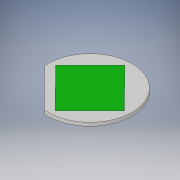
# Autodesk Inventor part: RockSat Plate
Saved by Autodesk Inventor 2017 (Build 210142000, 142)
## iProperties
Created: 2016-12-06
Part Number: RockSat Plate
Material: Generic
Document SubType Name: Modeling
Designer: qupec
Density: 1 g/cm^3
Appearance: Default
Author: qupec
Autodesk Inventor part; units mm, degrees
ref_plane "YZ Plane" through (0, 0, 0) normal (1, 0, 0) x (0, 1, 0)
ref_plane "XZ Plane" through (0, 0, 0) normal (0, 1, 0) x (-1, 0, 0)
ref_plane "XY Plane" through (0, 0, 0) normal (0, 0, 1) x (1, 0, 0)
sketch "Sketch1" plane through (0, 0, 0) normal (0, 1, 0) x (-1, 0, 0)
  arc A0 (13.4296, 151.8071) -> (151.8071, 13.4296) centre (0, 0) ccw
  line L0 (151.8071, 13.4296) -> (13.4296, 151.8071)
  dimension "d0" = 304.8
  dimension "d1" = 116.84
  constraints: 2 end point, 2 point on circle, 1 centre point, 1 coincident
  measures "d0" diameter of A0
  measures "d1" distance from line of point (0, 0) L0
extrude "Extrusion1" add sketch "Sketch1" along normal blind 12.7
sketch "Sketch2" plane through (0, 12.7, 0) normal (0, 1, 0) x (1, 0, 0)
  line L0 (-134.6862, 9.2408) -> (8.7197, -134.721)
  line L1 (8.7197, -134.721) -> (134.6862, -9.2408)
  line L2 (134.6862, -9.2408) -> (-8.7197, 134.721)
  line L3 (-8.7197, 134.721) -> (-134.6862, 9.2408)
  point P0 (0, 0)
  dimension "d4" = 203.2
  dimension "d5" = 177.8
  dimension "d6" = 88.9
  dimension "d7" = 101.6
  constraints: 8 end point, 3 perpendicular
  measures "d4" distance between parallel lines of L1 L3
  measures "d5" distance between parallel lines of L2 L0
  measures "d6" distance from line of point (0, 0) L2
  measures "d7" distance from line of point (0, 0) L1
extrude "Extrusion4" cut sketch "Sketch2" against normal blind 0.0025
equation "\"d6\" = 0.5 * d5"
equation "\"d7\" = 0.5 * d4"
body "Solid1"
